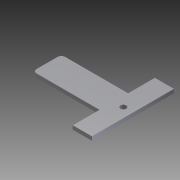
# Autodesk Inventor part: cetakan sepatu 4
Saved by Autodesk Inventor 2012 (Build 160160000, 160)
## iProperties
Created: 2014-01-20
Part Number: cetakan sepatu 4
Material: Default
Document SubType Name: Modeling
Designer: Irwan Haryanto
Density: 1 g/cm^3
Author: Irwan Haryanto
Autodesk Inventor part; units mm, degrees
ref_plane "YZ Plane" through (0, 0, 0) normal (1, 0, 0) x (0, 1, 0)
ref_plane "XZ Plane" through (0, 0, 0) normal (0, 1, 0) x (-1, 0, 0)
ref_plane "XY Plane" through (0, 0, 0) normal (0, 0, 1) x (1, 0, 0)
sketch "Sketch1" plane through (0, 0, 0) normal (0, 0, 1) x (1, 0, 0)
  line L0 (-29.3667, -90.0273) -> (-29.3667, -79.0273)
  arc A0 (-27.3667, -77.0273) -> (-29.3667, -79.0273) centre (-27.3667, -79.0273) ccw
  arc A1 (-29.3667, -90.0273) -> (-27.3667, -92.0273) centre (-27.3667, -90.0273) ccw
  line L1 (-27.3667, -77.0273) -> (5.5848, -77.0273)
  line L2 (-27.3667, -92.0273) -> (5.6333, -92.0273)
  line L3 (5.5848, -77.0273) -> (5.5848, -63.0273)
  line L4 (5.5848, -63.0273) -> (15.5848, -63.0273)
  line L5 (15.5848, -63.0273) -> (15.6333, -106.0273)
  line L6 (15.6333, -106.0273) -> (5.6333, -106.0273)
  line L7 (5.6333, -106.0273) -> (5.6333, -92.0273)
  circle A2 centre (10.609, -84.5273) radius 1.5
  point P0 (0, 0)
  dimension "d0" = 35
  dimension "d1" = 2
  dimension "d2" = 10
  dimension "d3" = 43
  dimension "d4" = 10
  dimension "d5" = 14
  dimension "d6" = 14
  dimension "d7" = 3
  dimension "d8" = 5
  dimension "d9" = 21.5
  constraints: 16 end point, 4 point on circle, 4 tangent, 3 centre point, 3 parallel, 2 perpendicular, 1 equal radius
  measures "d0" distance from line of L0 L7.end
  measures "d1" radius of A0
  measures "d2" distance of L4.start L5.start
  measures "d3" distance of L5.start L5.end
  measures "d4" distance of L5.end L6.end
  measures "d5" distance of L6.end L7.end
  measures "d6" distance of L3.start L4.start
  measures "d7" diameter of A2
  measures "d8" distance from line of L5 A2.centre
  measures "d9" distance from line of L4 A2.centre
extrude "Extrusion1" add sketch "Sketch1" along normal blind 2
body "Solid1"
